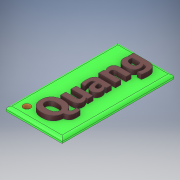
# Autodesk Inventor part: 3d print
Saved by Autodesk Inventor 2017 (Build 210142000, 142)
## iProperties
Created: 2019-02-08
Part Number: 3d print
Material: Generic
Document SubType Name: Sheet Metal
Designer: qthuynh
Density: 1 g/cm^3
Appearance: Default
Sheet Metal Rule: Default
Author: qthuynh
Autodesk Inventor part; units mm, degrees
ref_plane "YZ Plane" through (0, 0, 0) normal (1, 0, 0) x (0, 1, 0)
ref_plane "XZ Plane" through (0, 0, 0) normal (0, 1, 0) x (-1, 0, 0)
ref_plane "XY Plane" through (0, 0, 0) normal (0, 0, 1) x (1, 0, 0)
sketch "Sketch1" plane through (0, 0, 0) normal (0, 1, 0) x (-1, 0, 0)
  line L0 (0, 0) -> (25.4, 0)
  line L1 (25.4, 0) -> (25.4, -50.8)
  line L2 (25.4, -50.8) -> (0, -50.8)
  line L3 (0, -50.8) -> (0, 0)
  dimension "d0" = 25.4
  dimension "d1" = 50.8
  constraints: 8 end point, 2 parallel, 1 horizontal, 1 perpendicular
  measures "d0" distance of L1.end L2.end
  measures "d1" distance of L0.end L1.end
extrude "Extrusion1" add sketch "Sketch1" along normal blind 2.032
fillet "Fillet1" radius 1.27 4 edges at (-12.7, 2.032, 0) (-25.4, 2.032, -25.4) (-12.7, 2.032, -50.8) (0, 2.032, -25.4)
sketch "Sketch5" plane through (0, 2.032, 0) normal (0, 1, 0) x (1, 0, 0)
  point P0 (0, 0)
  point P1 (-20.563, 4.5696)
hole "Hole1" at (-20.563, 2.032, -4.5696) direction (0, -1, 0) diameter 3.175 depth 6.35 tip angle 118
sketch "Sketch6" plane through (0, 2.032, 0) normal (0, 1, 0) x (1, 0, 0)
  line L0 (-18.0831, 3.0273) -> (-18.0831, 48.8297) construction
  line L1 (-18.0831, 48.8297) -> (-4.8274, 48.8297) construction
  line L2 (-4.8274, 48.8297) -> (-4.8274, 3.0273) construction
  line L3 (-4.8274, 3.0273) -> (-18.0831, 3.0273) construction
  spline S0 degree 2 poles (-5.025, 13.3108) (-4.9262, 12.8991) (-4.8274, 12.0758) (-4.8274, 11.1948) knots 0 0 0 1 2 2 2
  spline S1 degree 2 poles (-4.8274, 11.1948) (-4.8274, 10.3962) (-5.2308, 9.2682) (-5.6013, 8.8895) knots 0 0 0 1 2 2 2
  spline S2 degree 2 poles (-5.6013, 8.8895) (-5.9636, 8.519) (-6.9516, 8.1403) (-7.5279, 8.1156) knots 0 0 0 1 2 2 2
  spline S3 degree 2 poles (-7.5279, 8.1156) (-7.6267, 5.9666) (-10.4179, 3.4884) (-12.7891, 3.4884) knots 0 0 0 1 2 2 2
  spline S4 degree 2 poles (-12.7891, 3.4884) (-15.2344, 3.4884) (-18.0831, 6.1066) (-18.0831, 8.4037) knots 0 0 0 1 2 2 2
  spline S5 degree 2 poles (-18.0831, 8.4037) (-18.0831, 10.6926) (-15.2509, 13.3273) (-12.7891, 13.3273) knots 0 0 0 1 2 2 2
  spline S6 degree 2 poles (-12.7891, 13.3273) (-10.9942, 13.3273) (-8.4254, 11.837) (-7.882, 10.4703) knots 0 0 0 1 2 2 2
  spline S7 degree 2 poles (-7.882, 10.4703) (-7.1327, 10.4868) (-6.5646, 11.1207) (-6.5646, 11.9111) knots 0 0 0 1 2 2 2
  spline S8 degree 2 poles (-6.5646, 11.9111) (-6.5646, 12.224) (-6.7458, 12.9074) (-6.8281, 13.0556) knots 0 0 0 1 2 2 2
  line L4 (-6.8281, 13.0556) -> (-6.8281, 13.3108)
  line L5 (-6.8281, 13.3108) -> (-5.025, 13.3108)
  spline S9 degree 2 poles (-10.2203, 10.0092) (-10.6649, 10.3386) (-11.8422, 10.6926) (-12.7973, 10.6926) knots 0 0 0 1 2 2 2
  spline S10 degree 2 poles (-12.7973, 10.6926) (-13.703, 10.6926) (-14.9792, 10.3221) (-15.3908, 10.001) knots 0 0 0 1 2 2 2
  spline S11 degree 2 poles (-15.3908, 10.001) (-15.8025, 9.6799) (-16.1648, 8.8566) (-16.1648, 8.412) knots 0 0 0 1 2 2 2
  spline S12 degree 2 poles (-16.1648, 8.412) (-16.1648, 7.9426) (-15.8272, 7.1769) (-15.3991, 6.8229) knots 0 0 0 1 2 2 2
  spline S13 degree 2 poles (-15.3991, 6.8229) (-15.0039, 6.51) (-13.6947, 6.1231) (-12.7891, 6.1231) knots 0 0 0 1 2 2 2
  spline S14 degree 2 poles (-12.7891, 6.1231) (-11.8587, 6.1231) (-10.6237, 6.4936) (-10.2038, 6.8147) knots 0 0 0 1 2 2 2
  spline S15 degree 2 poles (-10.2038, 6.8147) (-9.7839, 7.1358) (-9.4216, 7.9673) (-9.4216, 8.412) knots 0 0 0 1 2 2 2
  spline S16 degree 2 poles (-9.4216, 8.412) (-9.4216, 8.8648) (-9.8086, 9.7046) (-10.2203, 10.0092) knots 0 0 0 1 2 2 2
  line L6 (-7.7091, 21.8159) -> (-7.7091, 19.4282)
  line L7 (-7.7091, 19.4282) -> (-8.5571, 19.4282)
  spline S17 degree 2 poles (-8.5571, 19.4282) (-8.0384, 18.8107) (-7.495, 17.7733) (-7.495, 17.057) knots 0 0 0 1 2 2 2
  spline S18 degree 2 poles (-7.495, 17.057) (-7.495, 15.9208) (-8.9359, 14.6446) (-10.3849, 14.6446) knots 0 0 0 1 2 2 2
  line L8 (-10.3849, 14.6446) -> (-15.3744, 14.6446)
  line L9 (-15.3744, 14.6446) -> (-15.3744, 17.0488)
  line L10 (-15.3744, 17.0488) -> (-11.5705, 17.0488)
  spline S19 degree 2 poles (-11.5705, 17.0488) (-10.9777, 17.0488) (-10.2203, 17.1064) (-9.965, 17.2217) knots 0 0 0 1 2 2 2
  spline S20 degree 2 poles (-9.965, 17.2217) (-9.7263, 17.3369) (-9.4793, 17.7898) (-9.4793, 18.2015) knots 0 0 0 1 2 2 2
  spline S21 degree 2 poles (-9.4793, 18.2015) (-9.4793, 18.4485) (-9.7263, 19.1401) (-9.9403, 19.4282) knots 0 0 0 1 2 2 2
  line L11 (-9.9403, 19.4282) -> (-15.3744, 19.4282)
  line L12 (-15.3744, 19.4282) -> (-15.3744, 21.8159)
  line L13 (-15.3744, 21.8159) -> (-7.7091, 21.8159)
  spline S22 degree 2 poles (-8.5242, 27.8674) (-8.3183, 27.6204) (-7.989, 27.2335) (-7.8243, 26.9041) knots 0 0 0 1 2 2 2
  spline S23 degree 2 poles (-7.8243, 26.9041) (-7.6679, 26.583) (-7.5032, 25.9738) (-7.5032, 25.4304) knots 0 0 0 1 2 2 2
  spline S24 degree 2 poles (-7.5032, 25.4304) (-7.5032, 24.4094) (-8.87, 23.0674) (-9.9074, 23.0674) knots 0 0 0 1 2 2 2
  spline S25 degree 2 poles (-9.9074, 23.0674) (-10.7554, 23.0674) (-11.8093, 23.7508) (-12.1139, 24.393) knots 0 0 0 1 2 2 2
  spline S26 degree 2 poles (-12.1139, 24.393) (-12.4268, 25.0434) (-12.6738, 26.8465) (-12.7397, 27.8839) knots 0 0 0 1 2 2 2
  line L14 (-12.7397, 27.8839) -> (-12.7808, 27.8839)
  spline S27 degree 2 poles (-12.7808, 27.8839) (-13.4148, 27.8839) (-13.9006, 26.9453) (-13.9006, 26.0067) knots 0 0 0 1 2 2 2
  spline S28 degree 2 poles (-13.9006, 26.0067) (-13.9006, 25.5868) (-13.5959, 24.4506) (-13.3572, 23.9154) knots 0 0 0 1 2 2 2
  line L15 (-13.3572, 23.9154) -> (-13.3572, 23.7096)
  line L16 (-13.3572, 23.7096) -> (-15.2097, 23.7096)
  spline S29 degree 2 poles (-15.2097, 23.7096) (-15.3085, 24.0636) (-15.5884, 25.6444) (-15.5884, 26.4513) knots 0 0 0 1 2 2 2
  spline S30 degree 2 poles (-15.5884, 26.4513) (-15.5884, 28.4273) (-14.2711, 30.2387) (-12.9208, 30.2387) knots 0 0 0 1 2 2 2
  line L17 (-12.9208, 30.2387) -> (-7.7091, 30.2387)
  line L18 (-7.7091, 30.2387) -> (-7.7091, 27.8674)
  line L19 (-7.7091, 27.8674) -> (-8.5242, 27.8674)
  line L20 (-9.7098, 27.8674) -> (-11.2988, 27.8674)
  spline S31 degree 2 poles (-11.2988, 27.8674) (-11.2412, 27.2582) (-11.1506, 26.5089) (-11.0189, 26.1467) knots 0 0 0 1 2 2 2
  spline S32 degree 2 poles (-11.0189, 26.1467) (-10.9119, 25.8256) (-10.4673, 25.4798) (-10.105, 25.4798) knots 0 0 0 1 2 2 2
  spline S33 degree 2 poles (-10.105, 25.4798) (-9.5698, 25.4798) (-9.1664, 26.0643) (-9.1664, 26.6324) knots 0 0 0 1 2 2 2
  spline S34 degree 2 poles (-9.1664, 26.6324) (-9.1664, 26.9453) (-9.4546, 27.604) (-9.7098, 27.8674) knots 0 0 0 1 2 2 2
  line L21 (-7.7091, 39.1801) -> (-7.7091, 36.776)
  line L22 (-7.7091, 36.776) -> (-11.5047, 36.776)
  spline S35 degree 2 poles (-11.5047, 36.776) (-11.974, 36.776) (-12.8961, 36.7019) (-13.1102, 36.6031) knots 0 0 0 1 2 2 2
  spline S36 degree 2 poles (-13.1102, 36.6031) (-13.3736, 36.4796) (-13.5959, 36.0185) (-13.5959, 35.6233) knots 0 0 0 1 2 2 2
  spline S37 degree 2 poles (-13.5959, 35.6233) (-13.5959, 35.3351) (-13.3736, 34.7341) (-13.1349, 34.3965) knots 0 0 0 1 2 2 2
  line L23 (-13.1349, 34.3965) -> (-7.7091, 34.3965)
  line L24 (-7.7091, 34.3965) -> (-7.7091, 32.0088)
  line L25 (-7.7091, 32.0088) -> (-15.3744, 32.0088)
  line L26 (-15.3744, 32.0088) -> (-15.3744, 34.3965)
  line L27 (-15.3744, 34.3965) -> (-14.5263, 34.3965)
  spline S38 degree 2 poles (-14.5263, 34.3965) (-15.0203, 34.9811) (-15.5802, 36.0926) (-15.5802, 36.7677) knots 0 0 0 1 2 2 2
  spline S39 degree 2 poles (-15.5802, 36.7677) (-15.5802, 37.9369) (-14.0982, 39.1801) (-12.6985, 39.1801) knots 0 0 0 1 2 2 2
  line L28 (-12.6985, 39.1801) -> (-7.7091, 39.1801)
  spline S40 degree 2 poles (-8.59, 47.9157) (-7.5279, 47.9157) (-6.0377, 47.2982) (-5.626, 46.7713) knots 0 0 0 1 2 2 2
  spline S41 degree 2 poles (-5.626, 46.7713) (-5.2061, 46.2361) (-4.8274, 44.7541) (-4.8274, 43.8485) knots 0 0 0 1 2 2 2
  spline S42 degree 2 poles (-4.8274, 43.8485) (-4.8274, 43.0827) (-5.025, 41.7078) (-5.1567, 41.2055) knots 0 0 0 1 2 2 2
  line L29 (-5.1567, 41.2055) -> (-7.0751, 41.2055)
  line L30 (-7.0751, 41.2055) -> (-7.0751, 41.4855)
  spline S43 degree 2 poles (-7.0751, 41.4855) (-7.0092, 41.6584) (-6.8446, 42.1441) (-6.7787, 42.3911) knots 0 0 0 1 2 2 2
  spline S44 degree 2 poles (-6.7787, 42.3911) (-6.7046, 42.6875) (-6.6058, 43.2474) (-6.6058, 43.5356) knots 0 0 0 1 2 2 2
  spline S45 degree 2 poles (-6.6058, 43.5356) (-6.6058, 44.1449) (-6.8528, 44.9517) (-7.0833, 45.1576) knots 0 0 0 1 2 2 2
  spline S46 degree 2 poles (-7.0833, 45.1576) (-7.3221, 45.3634) (-7.9643, 45.5281) (-8.4583, 45.5281) knots 0 0 0 1 2 2 2
  line L31 (-8.4583, 45.5281) -> (-8.5983, 45.5281)
  spline S47 degree 2 poles (-8.5983, 45.5281) (-8.2442, 45.1246) (-7.8161, 44.0708) (-7.8161, 43.5109) knots 0 0 0 1 2 2 2
  spline S48 degree 2 poles (-7.8161, 43.5109) (-7.8161, 42.0206) (-9.751, 40.4069) (-11.7352, 40.4069) knots 0 0 0 1 2 2 2
  spline S49 degree 2 poles (-11.7352, 40.4069) (-12.6326, 40.4069) (-14.0653, 40.9009) (-14.5675, 41.3455) knots 0 0 0 1 2 2 2
  spline S50 degree 2 poles (-14.5675, 41.3455) (-15.0533, 41.7736) (-15.5802, 42.9675) (-15.5802, 43.6179) knots 0 0 0 1 2 2 2
  spline S51 degree 2 poles (-15.5802, 43.6179) (-15.5802, 44.2025) (-15.2838, 45.1329) (-15.0368, 45.5116) knots 0 0 0 1 2 2 2
  line L32 (-15.0368, 45.5116) -> (-15.3744, 45.6022)
  line L33 (-15.3744, 45.6022) -> (-15.3744, 47.9157)
  line L34 (-15.3744, 47.9157) -> (-8.59, 47.9157)
  line L35 (-10.1215, 45.5281) -> (-13.5959, 45.5281)
  spline S52 degree 2 poles (-13.5959, 45.5281) (-13.6783, 45.3552) (-13.7853, 44.8365) (-13.7853, 44.573) knots 0 0 0 1 2 2 2
  spline S53 degree 2 poles (-13.7853, 44.573) (-13.7853, 43.7167) (-12.6738, 42.8522) (-11.6776, 42.8522) knots 0 0 0 1 2 2 2
  spline S54 degree 2 poles (-11.6776, 42.8522) (-11.1836, 42.8522) (-10.492, 42.9839) (-10.2285, 43.1568) knots 0 0 0 1 2 2 2
  spline S55 degree 2 poles (-10.2285, 43.1568) (-9.965, 43.3297) (-9.7016, 43.8814) (-9.7016, 44.3095) knots 0 0 0 1 2 2 2
  spline S56 degree 2 poles (-9.7016, 44.3095) (-9.7016, 44.6306) (-9.9239, 45.2481) (-10.1215, 45.5281) knots 0 0 0 1 2 2 2
  point P0 (0, 0)
  constraints: 2 other
extrude "Extrusion3" add sketch "Sketch6" along normal blind 2.032
equation "\"BendRadius\" = Thickness"
equation "\"BendReliefWidth\" = Thickness"
equation "\"BendReliefDepth\" = 0.5 * Thickness"
equation "\"CornerReliefSize\" = 4 * Thickness"
equation "\"MinimumRemnant\" = 2 * Thickness"
equation "\"TransitionRadius\" = BendRadius"
equation "\"JacobiRadiusSize\" = Thickness"
equation "\"GapSize\" = Thickness"
equation "\"Thickness\" = 3.048"
body "Solid1"
